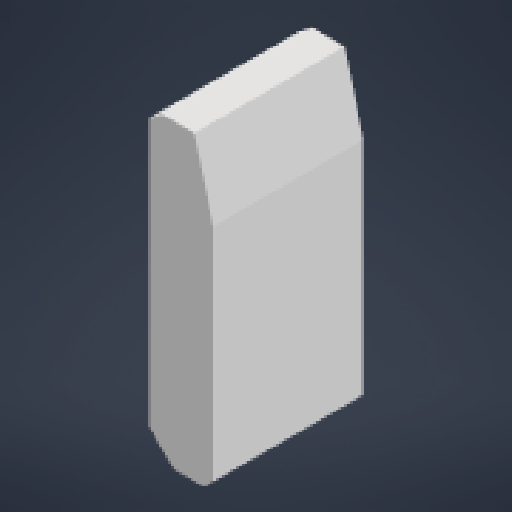
# Autodesk Inventor part: Тело
Saved by Autodesk Inventor 2026 (Build 300175000, 175)
## iProperties
Created: 2026-04-19
Part Number: Тело
Material: Типовые
Document SubType Name: Modeling
Designer: Artem Sannikov
Density: 1 g/cm^3
Appearance: По умолчанию
Author: Artem Sannikov
Autodesk Inventor part; units mm, degrees
ref_plane "YZ Plane" through (0, 0, 0) normal (1, 0, 0) x (0, 1, 0)
ref_plane "XZ Plane" through (0, 0, 0) normal (0, 1, 0) x (-1, 0, 0)
ref_plane "XY Plane" through (0, 0, 0) normal (0, 0, 1) x (1, 0, 0)
sketch "Эскиз1" plane through (0, 0, 0) normal (0, 0, 1) x (1, 0, 0)
  line L0 (29.9018, -80.1068) -> (83.774, -134.8208)
  line L1 (83.774, -134.8208) -> (164.0232, -134.8208)
  line L2 (164.0232, -134.8208) -> (202.5632, -96.8737)
  line L3 (202.5632, -96.8737) -> (202.5632, 92.1914)
  line L4 (202.5632, 92.1914) -> (202.5632, 579.95)
  line L5 (202.5632, 579.95) -> (189.081, 631.379)
  line L6 (189.081, 631.379) -> (87.3973, 631.379)
  line L7 (87.3973, 631.379) -> (29.9018, 588.3315)
  line L8 (29.9018, 588.3315) -> (29.9018, -80.1068)
  point P0 (0, 0)
  constraints: 18 end point, 3 perpendicular, 2 horizontal, 1 point on line
extrude "Выдавливание1" add sketch "Эскиз1" along normal blind 400
sketch "Эскиз2" plane through (0, 0, 0) normal (0, 0, -1) x (-1, 0, 0)
  circle A0 centre (-117.324, -35.3961) radius 10
  circle A1 centre (-117.324, 576.1543) radius 10
  point P0 (0, 0)
  dimension "d2" = 20
  dimension "d3" = 20
  constraints: 2 centre point
  measures "d2" diameter of A0
  measures "d3" diameter of A1
extrude "Выдавливание2" cut sketch "Эскиз2" against normal through all
